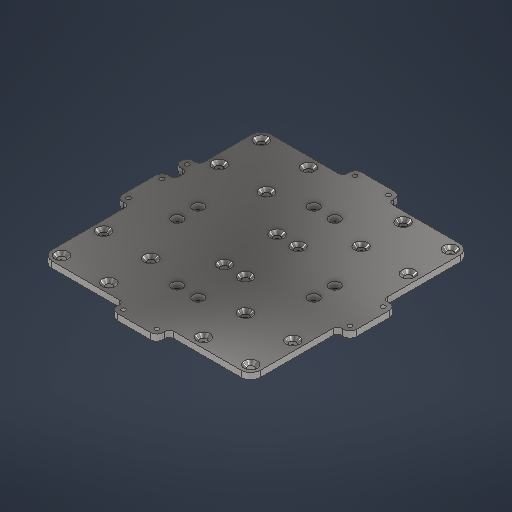
# Autodesk Inventor part: CNC-006-XAxisMount2
Saved by Autodesk Inventor 2026.2 (Build 302298000, 298)
## iProperties
Created: 2026-06-15
Part Number: CNC-006-XAxisMount2
Material: Steel AISI 1008 91 HR
Document SubType Name: Modeling
Designer: Kenji
Density: 7.872 g/cm^3
Appearance: Steel - Polished
Mass: 998.942 g
Surface Area: 598.243 cm^2
Volume: 126.898 cm^3
Author: Kenji
Autodesk Inventor part; units mm, degrees
ref_plane "YZ Plane" through (0, 0, 0) normal (1, 0, 0) x (0, 1, 0)
ref_plane "XZ Plane" through (0, 0, 0) normal (0, 1, 0) x (-1, 0, 0)
ref_plane "XY Plane" through (0, 0, 0) normal (0, 0, 1) x (1, 0, 0)
sketch "Sketch1" plane through (0, 0, 0) normal (0, 1, 0) x (-1, 0, 0)
  line L0 (-20, 26) -> (20, 26) construction
  line L1 (20, 26) -> (20, -26) construction
  line L2 (20, -26) -> (-20, -26) construction
  line L3 (-20, -26) -> (-20, 26) construction
  line L4 (-20, 26) -> (20, -26) construction
  line L5 (20, 26) -> (-20, -26) construction
  circle A0 centre (4, 20) radius 2.6
  circle A1 centre (-12, 20) radius 2.6
  circle A2 centre (4, -20) radius 2.6
  circle A3 centre (-12, -20) radius 2.6
  circle A4 centre (36, 44) radius 2.6
  circle A5 centre (36, 76) radius 2.6
  circle A6 centre (72, 76) radius 2.6
  circle A7 centre (72, 44) radius 2.6
  circle A8 centre (36, -44) radius 2.6
  circle A9 centre (72, -44) radius 2.6
  circle A10 centre (72, -76) radius 2.6
  circle A11 centre (36, -76) radius 2.6
  circle A12 centre (-36, 44) radius 2.6
  circle A13 centre (-36, 76) radius 2.6
  circle A14 centre (-72, 76) radius 2.6
  circle A15 centre (-72, 44) radius 2.6
  circle A16 centre (-36, -44) radius 2.6
  circle A17 centre (-36, -76) radius 2.6
  circle A18 centre (-72, -44) radius 2.6
  circle A19 centre (-72, -76) radius 2.6
  circle A20 centre (51.9938, 8.001) radius 4.1
  circle A21 centre (51.9938, -8.001) radius 4.1
  line L6 (0, -26) -> (0, 26) construction
  line L7 (20, 0) -> (-20, 0) construction
  circle A22 centre (8.001, 51.9938) radius 4.1
  circle A23 centre (-8.001, 51.9938) radius 4.1
  circle A24 centre (72, 76) radius 7.3625 construction
  circle A25 centre (72, -76) radius 7.3625 construction
  circle A26 centre (-72, -76) radius 7.3625 construction
  circle A27 centre (-72, 76) radius 7.3625 construction
  line L8 (79.3625, 76) -> (79.3625, -76)
  line L9 (72, -83.3625) -> (-72, -83.3625)
  line L10 (-79.3625, -76) -> (-79.3625, 76)
  line L11 (-72, 83.3625) -> (72, 83.3625)
  arc A28 (72, -83.3625) -> (79.3625, -76) centre (72, -76) ccw
  arc A29 (-79.3625, -76) -> (-72, -83.3625) centre (-72, -76) ccw
  arc A30 (-72, 83.3625) -> (-79.3625, 76) centre (-72, 76) ccw
  arc A31 (79.3625, 76) -> (72, 83.3625) centre (72, 76) ccw
  circle A32 centre (8.001, -51.9938) radius 4.1
  circle A33 centre (-8.001, -51.9938) radius 4.1
  circle A34 centre (-51.9938, 8.001) radius 4.1
  circle A35 centre (-51.9938, -8.001) radius 4.1
  point P0 (0, 0)
  point P1 (0, 0)
  point P2 (0, 0)
  point P3 (0, 0)
  dimension "d0" = 40
  dimension "d1" = 52
  dimension "d2" = 5.2
  dimension "d3" = 6
  dimension "d4" = 6
  dimension "d5" = 8
  dimension "d6" = 16
  dimension "d8" = 24
  dimension "d9" = 32
  dimension "d10" = 32
  dimension "d11" = 36
  dimension "d12" = 32
  dimension "d13" = 24
  dimension "d14" = 36
  dimension "d15" = 24
  dimension "d16" = 8.2
  dimension "d17" = 8.001
  dimension "d18" = 51.9938
  dimension "d19" = 8.001
  dimension "d20" = 8.001
  dimension "d21" = 8.001
  dimension "d22" = 51.9938
  dimension "d23" = 4.7625
  dimension "d27" = 51.9938
  dimension "d28" = 51.9938
  constraints: 36 centre point, 32 equal radius, 24 end point, 18 horizontal alignment, 18 vertical alignment, 16 point on circle, 8 midpoint, 7 tangent, 4 coincident, 3 perpendicular, 2 parallel, 1 horizontal
  measures "d0" distance between parallel lines of L3 L1
  measures "d1" distance between parallel lines of L2 L0
  measures "d2" diameter of A2
  measures "d3" distance from line of L0 A1.centre
  measures "d4" distance from line of L2 A3.centre
  measures "d5" distance from line of L3 A1.centre
  measures "d6" distance of A1.centre A0.centre
  measures "d8" vertical distance of A4.centre A0.centre
  measures "d9" horizontal distance of A0.centre A4.centre
  measures "d10" distance of A5.centre A4.centre
  measures "d11" distance of A5.centre A6.centre
  measures "d12" distance of A11.centre A8.centre
  measures "d13" vertical distance of A2.centre A8.centre
  measures "d14" distance of A14.centre A13.centre
  measures "d15" horizontal distance of A12.centre A1.centre
  measures "d16" diameter of A20
  measures "d17" vertical distance of point (0, 0) A20.centre
  measures "d18" horizontal distance of point (0, 0) A20.centre
  measures "d19" vertical distance of point (0, 0) A21.centre
  measures "d20" horizontal distance of point (0, 0) A22.centre
  measures "d21" horizontal distance of A23.centre point (0, 0)
  measures "d22" vertical distance of point (0, 0) A22.centre
  measures "d23" radial gap between concentric circles of A24 A6
  measures "d27" vertical distance of A32.centre point (0, 0)
  measures "d28" horizontal distance of A34.centre point (0, 0)
extrude "Extrusion1" add sketch "Sketch1" along normal blind 4.7625 contours L8 A28 L9 A29 L10 A30 L11 A31 | A32 | A33 | A34 | A35
extrude "Extrusion2" cut sketch "Sketch1" along normal through all contours A32 | A33 | A34 | A35
sketch "Sketch2" plane through (0, 4.7625, 0) normal (0, 1, 0) x (1, 0, 0)
  circle A0 centre (51.9938, 8.001) radius 4.1 projected
  circle A1 centre (8.001, 51.9938) radius 4.1 projected
  circle A2 centre (51.9938, -8.001) radius 4.1 projected
  circle A3 centre (-8.001, 51.9938) radius 4.1 projected
  line L0 (79.3625, -76) -> (79.3625, 76) projected
  arc A4 (79.3625, 76) -> (72, 83.3625) centre (72, 76) ccw projected
  line L1 (72, 83.3625) -> (-72, 83.3625) projected
  arc A5 (-72, 83.3625) -> (-79.3625, 76) centre (-72, 76) ccw projected
  line L2 (-79.3625, 76) -> (-79.3625, -76) projected
  arc A6 (-79.3625, -76) -> (-72, -83.3625) centre (-72, -76) ccw projected
  line L3 (-72, -83.3625) -> (72, -83.3625) projected
  arc A7 (72, -83.3625) -> (79.3625, -76) centre (72, -76) ccw projected
  circle A8 centre (8.001, -51.9938) radius 4.1 projected
  circle A9 centre (-51.9938, 8.001) radius 4.1 projected
  circle A10 centre (72, 44) radius 2.6 projected
  circle A11 centre (36, 44) radius 2.6 projected
  circle A12 centre (36, -76) radius 2.6 projected
  circle A13 centre (-36, 76) radius 2.6 projected
  circle A14 centre (-36, 44) radius 2.6 projected
  circle A15 centre (-72, -44) radius 2.6 projected
  circle A16 centre (-36, -76) radius 2.6 projected
  circle A17 centre (-36, -44) radius 2.6 projected
  circle A18 centre (12, 20) radius 2.6 projected
  circle A19 centre (-4, 20) radius 2.6 projected
  circle A20 centre (12, -20) radius 2.6 projected
  circle A21 centre (-4, -20) radius 2.6 projected
  circle A22 centre (-72, 44) radius 2.6 projected
  circle A23 centre (36, -44) radius 2.6 projected
  circle A24 centre (72, -44) radius 2.6 projected
  circle A25 centre (36, 76) radius 2.6 projected
  circle A26 centre (-51.9938, -8.001) radius 4.1 projected
  circle A27 centre (-8.001, -51.9938) radius 4.1 projected
  circle A28 centre (72, 76) radius 2.6 projected
  circle A29 centre (72, -76) radius 2.6 projected
  circle A30 centre (-72, 76) radius 2.6 projected
  circle A31 centre (-72, -76) radius 2.6 projected
  point P0 (0, 0)
hole "Hole1" at (-72, 4.7625, 76) at (-72, 4.7625, 44) at (-36, 4.7625, 76) at (-36, 4.7625, 44) at (-4, 4.7625, 20) at (12, 4.7625, 20) at (-4, 4.7625, -20) at (12, 4.7625, -20) at (36, 4.7625, 44) at (36, 4.7625, 76) at (72, 4.7625, 76) at (72, 4.7625, 44) at (-72, 4.7625, -44) at (-72, 4.7625, -76) at (-36, 4.7625, -44) at (-36, 4.7625, -76) at (36, 4.7625, -76) at (36, 4.7625, -44) at (72, 4.7625, -44) at (72, 4.7625, -76) direction (0, -1, 0) diameter 4.019 end through all countersink diameter 10 countersink angle 90 thread size "M5" standard "Din Taper"
sketch "Sketch3" plane through (0, 4.7625, 0) normal (0, 1, 0) x (1, 0, 0)
  circle A0 centre (-12.7, -88.1875) radius 1.65
  line L0 (-72, -83.3625) -> (72, -83.3625) projected
  circle A1 centre (72, 76) radius 5 projected
  circle A2 centre (72, 44) radius 5 projected
  circle A3 centre (36, 44) radius 5 projected
  circle A4 centre (36, 76) radius 5 projected
  circle A5 centre (-36, 76) radius 5 projected
  circle A6 centre (-36, 44) radius 5 projected
  circle A7 centre (-72, 76) radius 5 projected
  circle A8 centre (-72, 44) radius 5 projected
  circle A9 centre (72, -44) radius 5 projected
  circle A10 centre (72, -76) radius 5 projected
  circle A11 centre (36, -76) radius 5 projected
  circle A12 centre (36, -44) radius 5 projected
  circle A13 centre (12, 20) radius 5 projected
  circle A14 centre (-4, 20) radius 5 projected
  circle A15 centre (12, -20) radius 5 projected
  circle A16 centre (-4, -20) radius 5 projected
  circle A17 centre (-36, -44) radius 5 projected
  circle A18 centre (-36, -76) radius 5 projected
  circle A19 centre (-72, -44) radius 5 projected
  circle A20 centre (-72, -76) radius 5 projected
  circle A21 centre (51.9938, 8.001) radius 4.1 projected
  circle A22 centre (8.001, 51.9938) radius 4.1 projected
  circle A23 centre (51.9938, -8.001) radius 4.1 projected
  circle A24 centre (-8.001, 51.9938) radius 4.1 projected
  line L1 (79.3625, -76) -> (79.3625, 76) projected
  arc A25 (79.3625, 76) -> (72, 83.3625) centre (72, 76) ccw projected
  line L2 (72, 83.3625) -> (-72, 83.3625) projected
  arc A26 (-72, 83.3625) -> (-79.3625, 76) centre (-72, 76) ccw projected
  line L3 (-79.3625, 76) -> (-79.3625, -76) projected
  arc A27 (-79.3625, -76) -> (-72, -83.3625) centre (-72, -76) ccw projected
  line L4 (-72, -83.3625) -> (72, -83.3625) projected
  arc A28 (72, -83.3625) -> (79.3625, -76) centre (72, -76) ccw projected
  circle A29 centre (8.001, -51.9938) radius 4.1 projected
  circle A30 centre (-51.9938, 8.001) radius 4.1 projected
  circle A31 centre (-51.9938, -8.001) radius 4.1 projected
  circle A32 centre (-8.001, -51.9938) radius 4.1 projected
  circle A33 centre (12.7, -88.1875) radius 1.65
  circle A34 centre (-12.7, -88.1875) radius 4.825 construction
  circle A35 centre (12.7, -88.1875) radius 4.825 construction
  circle A36 centre (-84.1875, -12.7) radius 1.65
  circle A37 centre (-84.1875, 12.7) radius 1.65
  circle A38 centre (-84.1875, -12.7) radius 4.825 construction
  circle A39 centre (-84.1875, 12.7) radius 4.825 construction
  circle A40 centre (84.1875, 12.7) radius 1.65
  circle A41 centre (84.1875, -12.7) radius 1.65
  circle A42 centre (84.1875, 12.7) radius 4.825 construction
  circle A43 centre (84.1875, -12.7) radius 4.825 construction
  circle A44 centre (-12.7, 88.1875) radius 4.825 construction
  circle A45 centre (12.7, 88.1875) radius 4.825 construction
  line L5 (72, 83.3625) -> (-72, 83.3625) construction
  circle A46 centre (-12.7, 88.1875) radius 1.65
  circle A47 centre (12.7, 88.1875) radius 1.65
  arc A48 (79.3625, 20.528) -> (83.1923, 17.4213) centre (82.5375, 20.528) ccw
  line L6 (79.3625, -76) -> (79.3625, 76) projected
  arc A49 (83.1923, -17.4213) -> (79.3625, -20.528) centre (82.5375, -20.528) ccw
  line L7 (89.0125, -12.7) -> (89.0125, 12.7)
  arc A50 (89.0125, 12.7) -> (83.1923, 17.4213) centre (84.1875, 12.7) ccw
  arc A51 (83.1923, -17.4213) -> (89.0125, -12.7) centre (84.1875, -12.7) ccw
  arc A52 (-20.528, 83.3625) -> (-17.4213, 87.1923) centre (-20.528, 86.5375) ccw
  arc A53 (17.4213, 87.1923) -> (20.528, 83.3625) centre (20.528, 86.5375) ccw
  line L8 (-12.7, 93.0125) -> (12.7, 93.0125)
  arc A54 (-12.7, 93.0125) -> (-17.4213, 87.1923) centre (-12.7, 88.1875) ccw
  arc A55 (17.4213, 87.1923) -> (12.7, 93.0125) centre (12.7, 88.1875) ccw
  arc A56 (-83.1923, 17.4213) -> (-79.3625, 20.528) centre (-82.5375, 20.528) ccw
  arc A57 (-79.3625, -20.528) -> (-83.1923, -17.4213) centre (-82.5375, -20.528) ccw
  line L9 (-89.0125, -12.7) -> (-89.0125, 12.7)
  arc A58 (-83.1923, 17.4213) -> (-89.0125, 12.7) centre (-84.1875, 12.7) ccw
  arc A59 (-89.0125, -12.7) -> (-83.1923, -17.4213) centre (-84.1875, -12.7) ccw
  arc A60 (-17.4213, -87.1923) -> (-20.528, -83.3625) centre (-20.528, -86.5375) ccw
  arc A61 (20.528, -83.3625) -> (17.4213, -87.1923) centre (20.528, -86.5375) ccw
  line L10 (-12.7, -93.0125) -> (12.7, -93.0125)
  arc A62 (-17.4213, -87.1923) -> (-12.7, -93.0125) centre (-12.7, -88.1875) ccw
  arc A63 (12.7, -93.0125) -> (17.4213, -87.1923) centre (12.7, -88.1875) ccw
  point P0 (0, 0)
  point P1 (-20.528, 83.3625)
  point P2 (20.528, -83.3625)
  point P3 (-20.528, -83.3625)
  dimension "d40" = 3.3
  dimension "d42" = 12.7
  dimension "d43" = 25.4
  dimension "d44" = 3.175
  dimension "d45" = 12.7
  dimension "d46" = 25.4
  dimension "d47" = 3.175
  constraints: 48 point on circle, 34 tangent, 32 centre point, 25 equal radius, 8 end point, 8 point on line, 7 coincident, 4 vertical alignment, 3 horizontal alignment, 2 vertical, 1 horizontal
  measures "d40" diameter of A0
  measures "d42" horizontal distance of A0.centre point (0, 0)
  measures "d43" distance of A33.centre A0.centre
  measures "d44" radial gap between concentric circles of A34 A0
  measures "d45" vertical distance of point (0, 0) A37.centre
  measures "d46" distance of A37.centre A36.centre
  measures "d47" radius of A48
extrude "Extrusion3" add sketch "Sketch3" against normal up to surface (4.7625 mm away) contours L0 A61 A63 L10 A62 A60 | A57 A59 L9 A58 A56 L3 | L1 A48 A50 L7 A51 A49 | A52 A54 L8 A55 A53 L2
sketch "Sketch4" plane through (0, 4.7625, 0) normal (0, 1, 0) x (1, 0, 0)
  circle A0 centre (-72, -76) radius 2.6 projected
  circle A1 centre (-36, -76) radius 2.6 projected
  line L0 (-79.3625, -20.528) -> (-79.3625, -76) construction
  circle A2 centre (-84.1875, -12.7) radius 1.65 projected
  line L1 (-79.3625, -39.9296) -> (-79.3625, -23.5598)
  line L2 (-79.3625, -20.528) -> (-79.3625, -76) projected
  circle A3 centre (84.1875, -12.7) radius 1.65 projected
  circle A4 centre (-84.1875, 31.75) radius 1.65
  circle A5 centre (-84.1875, 12.7) radius 1.65 projected
  circle A6 centre (-84.1875, 31.75) radius 4.825 construction
  line L3 (-79.3625, 76) -> (-79.3625, 20.528) projected
  arc A7 (-83.1923, 36.4713) -> (-79.3625, 39.578) centre (-82.5375, 39.578) ccw
  arc A8 (-79.3625, 23.922) -> (-83.1923, 27.0287) centre (-82.5375, 23.922) ccw
  arc A9 (-83.1923, 36.4713) -> (-82.9884, 27.0764) centre (-84.1875, 31.75) ccw
  circle A10 centre (-57.15, 88.1875) radius 1.65 construction
  circle A11 centre (-12.7, 88.1875) radius 1.65 projected
  circle A12 centre (-57.15, 88.1875) radius 4.825 construction
  line L4 (-20.528, 83.3625) -> (-72, 83.3625) construction
  arc A13 (-52.4287, 87.1923) -> (-49.322, 83.3625) centre (-49.322, 86.5375) ccw construction
  arc A14 (-64.978, 83.3625) -> (-61.8713, 87.1923) centre (-64.978, 86.5375) ccw construction
  arc A15 (-52.4287, 87.1923) -> (-61.8713, 87.1923) centre (-57.15, 88.1875) ccw construction
  line L5 (-64.978, 83.3625) -> (-49.322, 83.3625) construction
  point P0 (0, 0)
  point P1 (-83.1923, 27.0287)
  dimension "d71" = 3.3
  dimension "d72" = 19.05
  dimension "d73" = 3.175
  dimension "d74" = 3.175
  dimension "d75" = 44.45
  constraints: 17 point on circle, 12 tangent, 10 centre point, 6 equal radius, 6 point on line, 4 end point, 2 collinear, 1 coincident
  measures "d71" diameter of A4
  measures "d72" distance of A4.centre A5.centre
  measures "d73" radial gap between concentric circles of A6 A4
  measures "d74" radius of A7
  measures "d75" distance of A11.centre A10.centre
thread "Thread1" size "M4x0.7" class "6H" standard "ISO Metric profile" full length
thread "Thread2" size "M4x0.7" class "6H" standard "ISO Metric profile" full length
extrude "Extrusion6" add sketch "Sketch4" against normal up to surface (4.7625 mm away) contours L3 A8 A9 A7
thread "Thread3" size "M4x0.7" class "6H" standard "ISO Metric profile" full length
thread "Thread4" size "M4x0.7" class "6H" standard "ISO Metric profile" full length
equation "\"d4\" = d3"
equation "\"d12\" = d10"
equation "\"d13\" = d8"
equation "\"d14\" = d11"
equation "\"d17\" = d20"
equation "\"d19\" = d17"
equation "\"d21\" = d20"
equation "\"d22\" = d18"
equation "\"d27\" = d22"
equation "\"d28\" = d27"
equation "\"d45\" = d42"
equation "\"d46\" = d43"
body "Solid1"
